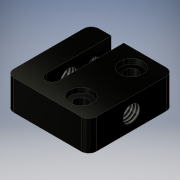
# Autodesk Inventor part: Anti-Backlash Nut Block
Saved by Autodesk Inventor 2019 (Build 230136000, 136)
## iProperties
Created: 2020-11-22
Part Number: Anti-Backlash Nut Block
Material: Aluminum 6061
Document SubType Name: Modeling
Designer: asus
Density: 2.7 g/cm^3
Appearance: Gunmetal
Author: asus
Autodesk Inventor part; units mm, degrees
ref_plane "YZ Plane" through (0, 0, 0) normal (1, 0, 0) x (0, 1, 0)
ref_plane "XZ Plane" through (0, 0, 0) normal (0, 1, 0) x (-1, 0, 0)
ref_plane "XY Plane" through (0, 0, 0) normal (0, 0, 1) x (1, 0, 0)
sketch "Sketch1" plane through (0, 0, 0) normal (0, 1, 0) x (-1, 0, 0)
  line L0 (13.46, 17) -> (-13.46, 17)
  line L1 (-16.5, 13.96) -> (-16.5, -13.96)
  line L2 (16.5, -13.96) -> (16.5, 13.96)
  line L3 (6, -19) -> (6, 9) construction
  line L4 (8.5, -17) -> (8.5, 9)
  line L5 (3.5, 9) -> (3.5, -17)
  arc A0 (8.5, 9) -> (3.5, 9) centre (6, 9) ccw
  circle A1 centre (-6.5, 10) radius 2.5
  circle A2 centre (-6.5, -10) radius 2.5
  line L6 (-13.46, -17) -> (3.5, -17)
  line L7 (8.5, -17) -> (13.46, -17)
  arc A3 (13.46, -17) -> (16.5, -13.96) centre (13.46, -13.96) ccw
  arc A4 (16.5, 13.96) -> (13.46, 17) centre (13.46, 13.96) ccw
  arc A5 (-13.46, 17) -> (-16.5, 13.96) centre (-13.46, 13.96) ccw
  arc A6 (-16.5, -13.96) -> (-13.46, -17) centre (-13.46, -13.96) ccw
  point P0 (0, 0)
  point P1 (-16.5, -17)
  point P2 (-16.5, 17)
  point P3 (16.5, -17)
  point P4 (16.5, 0)
  point P5 (0, -17)
  point P6 (6, -5)
  dimension "d0" = 33
  dimension "d1" = 34
  dimension "d2" = 5
  dimension "d4" = 28
  dimension "d5" = 8
  dimension "d6" = 5
  dimension "d7" = 5
  dimension "d8" = 20
  dimension "d9" = 10
  dimension "d10" = 7
  dimension "d11" = 3.04
  constraints: 18 end point, 10 point on circle, 10 tangent, 7 centre point, 7 point on line, 4 parallel, 3 equal radius, 2 horizontal alignment, 2 midpoint, 2 vertical alignment, 1 horizontal, 1 perpendicular, 1 vertical
  measures "d0" distance of point (16.5, -17) point (-16.5, -17)
  measures "d1" distance of point (-16.5, -17) point (-16.5, 17)
  measures "d2" diameter of A0
  measures "d4" distance of L3.start L3.end
  measures "d5" distance between parallel lines of L2 L4
  measures "d6" diameter of A1
  measures "d7" diameter of A2
  measures "d8" distance of A1.centre A2.centre
  measures "d9" distance from line of L1 A1.centre
  measures "d10" distance from line of L0 A1.centre
  measures "d11" radius of A3
extrude "Extrusion1" add sketch "Sketch1" along normal blind 12
sketch "Sketch2" plane through (-16.5, 0, -13.96) normal (-1, 0, 0) x (0, 0, 1)
  circle A0 centre (13.96, 6) radius 4
  circle A1 centre (3.96, 6) radius 2.5
  line L0 (0, 0) -> (27.92, 0) projected
  point P0 (13.96, 0)
  point P1 (13.96, 0)
  dimension "d14" = 8
  dimension "d15" = 5
  dimension "d16" = 6
  dimension "d17" = 10
  constraints: 2 centre point, 1 horizontal alignment, 1 midpoint, 1 vertical alignment
  measures "d14" diameter of A0
  measures "d15" diameter of A1
  measures "d16" distance from line of L0 A0.centre
  measures "d17" distance of A0.centre A1.centre
hole "Hole1" at (-16.5, 6, 0) direction (1, 0, 0) diameter 6.647 depth 40 tip angle 118 thread size "M8x1.25" class "6H" standard "ISO Metric profile"
hole "Hole2" at (-16.5, 6, -10) direction (1, 0, 0) diameter 4.134 depth 10 tip angle 118 thread size "M5x0.8" class "6H" standard "ISO Metric profile"
sketch "Sketch3" plane through (0, 12, 0) normal (0, 1, 0) x (1, 0, 0)
  circle A0 centre (6.5, 10) radius 2.5 projected
  circle A1 centre (6.5, -10) radius 2.5 projected
  circle A2 centre (6.5, 10) radius 4.5
  circle A3 centre (6.5, -10) radius 4.5
  point P0 (0, 0)
  dimension "d32" = 9
  dimension "d33" = 9
  constraints: 2 centre point, 2 coincident
  measures "d32" diameter of A2
  measures "d33" diameter of A3
extrude "Extrusion2" cut sketch "Sketch3" against normal blind 2
sketch "Sketch4" plane through (0, 0, 0) normal (0, -1, 0) x (1, 0, 0)
  circle A0 centre (6.5, 10) radius 2.5 projected
  circle A1 centre (6.5, -10) radius 2.5 projected
  line L0 (4.1906, 6) -> (1.8812, 10)
  line L1 (1.8812, 10) -> (4.1906, 14)
  line L2 (4.1906, 14) -> (8.8094, 14)
  line L3 (8.8094, 14) -> (11.1188, 10)
  line L4 (11.1188, 10) -> (8.8094, 6)
  line L5 (8.8094, 6) -> (4.1906, 6)
  line L6 (8.8094, -6) -> (11.1188, -10)
  line L7 (11.1188, -10) -> (8.8094, -14)
  line L8 (8.8094, -14) -> (4.1906, -14)
  line L9 (4.1906, -14) -> (1.8812, -10)
  line L10 (1.8812, -10) -> (4.1906, -6)
  line L11 (4.1906, -6) -> (8.8094, -6)
  point P0 (0, 0)
  dimension "d36" = 8
  dimension "d37" = 8
  constraints: 24 end point, 2 coincident, 26 other
  measures "d36" distance between parallel lines of L8 L11
  measures "d37" distance between parallel lines of L2 L5
extrude "Extrusion3" cut sketch "Sketch4" against normal blind 5
body "Solid1"
